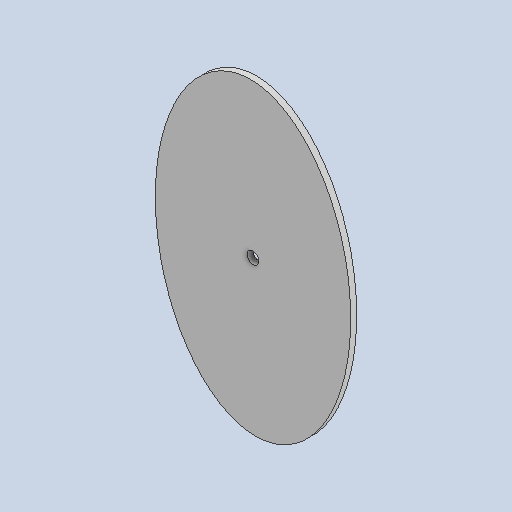
# Autodesk Inventor part: верхний эллипс туловища
Saved by Autodesk Inventor 2023.1 (Build 271208000, 208)
## iProperties
Created: 2024-11-21
Part Number: верхний эллипс туловища
Material: Типовые
Document SubType Name: Modeling
Designer: DELL
Density: 1 g/cm^3
Appearance: По умолчанию
Author: DELL
Autodesk Inventor part; units mm, degrees
ref_plane "YZ Plane" through (0, 0, 0) normal (1, 0, 0) x (0, 1, 0)
ref_plane "XZ Plane" through (0, 0, 0) normal (0, 1, 0) x (-1, 0, 0)
ref_plane "XY Plane" through (0, 0, 0) normal (0, 0, 1) x (1, 0, 0)
sketch "Эскиз1" plane through (0, 0, 0) normal (0, 0, 1) x (1, 0, 0)
  ellipse E0 centre (0, 0) end of major axis (2.8994, -101.9588) minor radius 65
  circle A0 centre (0, 0) radius 4
  dimension "d0" = 102
  dimension "d1" = 65
  dimension "d4" = 8
  constraints: 2 centre point, 2 coincident
  measures "d4" diameter of A0
extrude "Выдавливание1" add sketch "Эскиз1" against normal blind 4
